Autodesk Inventor part; units mm, degrees
(part 2 of 2)
  line L319 (-28.6263, 18.3241) -> (-28.6263, 16.0044)
  line L320 (-28.6263, 16.0044) -> (-25.6449, 16.0044)
  line L321 (-25.6449, 18.3241) -> (-28.6263, 18.3241)
  line L322 (-29.7503, 19.4482) -> (-24.5209, 19.4482)
  line L323 (-29.5884, 13.8513) -> (-27.9357, 13.8513)
  line L324 (-29.5884, 12.8808) -> (-29.5884, 13.8513)
  line L325 (-29.7503, 14.8804) -> (-29.7503, 19.4482)
  line L326 (-26.6942, 13.8513) -> (-19.7097, 13.8513)
  line L327 (-23.8, 11.9101) -> (-23.8, 12.8808)
  line L328 (-25.8364, 11.9101) -> (-23.8, 11.9101)
  line L329 (-24.7124, 10.786) -> (-24.7124, 8.4664)
  line L330 (-21.731, 8.4664) -> (-21.731, 10.786)
  line L331 (-24.7124, 8.4664) -> (-21.731, 8.4664)
  line L332 (-21.731, 10.786) -> (-24.7124, 10.786)
  line L333 (-26.6942, 14.8804) -> (-26.6942, 13.8513)
  line L334 (-24.5209, 14.8804) -> (-26.6942, 14.8804)
  line L335 (-20.607, 11.9101) -> (-20.607, 7.3423)
  line L336 (-20.607, 7.3423) -> (-25.8364, 7.3423)
  line L337 (-25.8364, 7.3423) -> (-25.8364, 11.9101)
  line L338 (-27.9357, 14.8804) -> (-29.7503, 14.8804)
  line L339 (-37.8438, 41.8417) -> (-37.8438, 39.522)
  line L340 (-41.854, 38.3672) -> (-47.0835, 38.3672)
  line L341 (-45.9594, 39.4913) -> (-42.9781, 39.4913)
  line L342 (-42.9781, 39.4913) -> (-42.9781, 41.8109)
  line L343 (-39.6887, 44.9654) -> (-33.9003, 44.9654)
  line L344 (-43.779, 42.935) -> (-41.854, 42.935)
  line L345 (-42.9781, 41.8109) -> (-45.9594, 41.8109)
  line L346 (-47.8027, 44.9654) -> (-40.8666, 44.9654)
  line L347 (-43.779, 43.9948) -> (-43.779, 42.935)
  line L348 (-44.8621, 42.935) -> (-44.8621, 43.9948)
  line L349 (-47.0835, 42.935) -> (-44.8621, 42.935)
  line L350 (-44.8621, 43.9948) -> (-47.8027, 43.9948)
  line L351 (-45.9594, 41.8109) -> (-45.9594, 39.4913)
  line L352 (-47.0835, 38.3672) -> (-47.0835, 42.935)
  line L353 (-35.553, 43.9948) -> (-35.553, 42.9657)
  line L354 (-40.8666, 44.9654) -> (-40.8666, 45.9361)
  line L355 (-41.854, 42.935) -> (-41.854, 38.3672)
  line L356 (-40.8666, 45.9361) -> (-42.8818, 45.9361)
  line L357 (-47.8027, 43.9948) -> (-47.8027, 44.9654)
  line L358 (-38.9678, 38.398) -> (-38.9678, 42.9657)
  line L359 (-34.8624, 39.522) -> (-34.8624, 41.8417)
  line L360 (-34.8624, 41.8417) -> (-37.8438, 41.8417)
  line L361 (-37.8438, 39.522) -> (-34.8624, 39.522)
  line L362 (-33.7384, 38.398) -> (-38.9678, 38.398)
  line L363 (-33.9003, 43.9948) -> (-35.553, 43.9948)
  line L364 (-33.9003, 44.9654) -> (-33.9003, 43.9948)
  line L365 (-33.7384, 42.9657) -> (-33.7384, 38.398)
  line L366 (-36.7945, 43.9948) -> (-43.779, 43.9948)
  line L367 (-39.6887, 45.9361) -> (-39.6887, 44.9654)
  line L368 (-37.6523, 45.9361) -> (-39.6887, 45.9361)
  line L369 (-38.7764, 47.0601) -> (-38.7764, 49.3798)
  line L370 (-41.7577, 49.3798) -> (-41.7577, 47.0601)
  line L371 (-38.7764, 49.3798) -> (-41.7577, 49.3798)
  line L372 (-41.7577, 47.0601) -> (-38.7764, 47.0601)
  line L373 (-36.7945, 42.9657) -> (-36.7945, 43.9948)
  line L374 (-38.9678, 42.9657) -> (-36.7945, 42.9657)
  line L375 (-42.8818, 45.9361) -> (-42.8818, 50.5038)
  line L376 (-42.8818, 50.5038) -> (-37.6523, 50.5038)
  line L377 (-37.6523, 50.5038) -> (-37.6523, 45.9361)
  line L378 (-35.553, 42.9657) -> (-33.7384, 42.9657)
  line L379 (-40.5846, 75.534) -> (-40.5846, 13.366) construction
  line L380 (-23.2199, 44.9654) -> (-23.2199, 45.9361)
  line L381 (-23.2199, 45.9361) -> (-25.235, 45.9361)
  line L382 (-19.1478, 43.9948) -> (-26.1323, 43.9948)
  line L383 (-24.111, 47.0601) -> (-21.1296, 47.0601)
  line L384 (-20.0056, 45.9361) -> (-22.042, 45.9361)
  line L385 (-24.111, 49.3798) -> (-24.111, 47.0601)
  line L386 (-25.235, 45.9361) -> (-25.235, 50.5038)
  line L387 (-21.1296, 47.0601) -> (-21.1296, 49.3798)
  line L388 (-21.1296, 49.3798) -> (-24.111, 49.3798)
  line L389 (-25.235, 50.5038) -> (-20.0056, 50.5038)
  line L390 (-20.0056, 50.5038) -> (-20.0056, 45.9361)
  line L391 (-22.042, 45.9361) -> (-22.042, 44.9654)
  line L392 (-24.2073, 38.3672) -> (-29.4368, 38.3672)
  line L393 (-28.3127, 39.4913) -> (-25.3314, 39.4913)
  line L394 (-25.3314, 39.4913) -> (-25.3314, 41.8109)
  line L395 (-26.1323, 42.935) -> (-24.2073, 42.935)
  line L396 (-25.3314, 41.8109) -> (-28.3127, 41.8109)
  line L397 (-30.156, 44.9654) -> (-23.2199, 44.9654)
  line L398 (-27.2154, 42.935) -> (-27.2154, 43.9948)
  line L399 (-30.156, 43.9948) -> (-30.156, 44.9654)
  line L400 (-27.2154, 43.9948) -> (-30.156, 43.9948)
  line L401 (-29.4368, 42.935) -> (-27.2154, 42.935)
  line L402 (-28.3127, 41.8109) -> (-28.3127, 39.4913)
  line L403 (-29.4368, 38.3672) -> (-29.4368, 42.935)
  line L404 (-26.1323, 43.9948) -> (-26.1323, 42.935)
  line L405 (-20.1971, 41.8417) -> (-20.1971, 39.522)
  line L406 (-22.042, 44.9654) -> (-16.2536, 44.9654)
  line L407 (-17.9063, 43.9948) -> (-17.9063, 42.9657)
  line L408 (-24.2073, 42.935) -> (-24.2073, 38.3672)
  line L409 (-21.3211, 38.398) -> (-21.3211, 42.9657)
  line L410 (-21.3211, 42.9657) -> (-19.1478, 42.9657)
  line L411 (-19.1478, 42.9657) -> (-19.1478, 43.9948)
  line L412 (-16.2536, 44.9654) -> (-16.2536, 43.9948)
  line L413 (-16.2536, 43.9948) -> (-17.9063, 43.9948)
  line L414 (-17.2157, 41.8417) -> (-20.1971, 41.8417)
  line L415 (-17.9063, 42.9657) -> (-16.0917, 42.9657)
  line L416 (-20.1971, 39.522) -> (-17.2157, 39.522)
  line L417 (-16.0917, 38.398) -> (-21.3211, 38.398)
  line L418 (-16.0917, 42.9657) -> (-16.0917, 38.398)
  line L419 (-17.2157, 39.522) -> (-17.2157, 41.8417)
  spline S0 degree 2 poles (-50.3948, 78.6019) (-50.3948, 77.8197) (-50.9135, 76.4941) (-51.3498, 76.0495) knots 0 0 0 1 2 2 2
  spline S1 degree 2 poles (-51.3498, 76.0495) (-51.8027, 75.5802) (-52.9389, 75.0945) (-53.6222, 75.0945) knots 0 0 0 1 2 2 2
  spline S2 degree 2 poles (-53.6222, 75.0945) (-54.3056, 75.0945) (-55.4336, 75.5555) (-55.8617, 76.0166) knots 0 0 0 1 2 2 2
  spline S3 degree 2 poles (-55.8617, 76.0166) (-56.3887, 76.5682) (-56.9815, 78.4207) (-56.9815, 79.771) knots 0 0 0 1 2 2 2
  spline S4 degree 2 poles (-56.9815, 79.771) (-56.9815, 81.0966) (-56.4381, 83.229) (-55.87, 84.0195) knots 0 0 0 1 2 2 2
  spline S5 degree 2 poles (-55.87, 84.0195) (-55.3183, 84.7934) (-53.5728, 85.6579) (-52.4284, 85.6579) knots 0 0 0 1 2 2 2
  spline S6 degree 2 poles (-52.4284, 85.6579) (-52.0908, 85.6579) (-51.498, 85.592) (-51.2757, 85.5179) knots 0 0 0 1 2 2 2
  line L420 (-51.2757, 85.5179) -> (-51.2757, 84.2088)
  line L421 (-51.2757, 84.2088) -> (-51.3334, 84.2088)
  spline S7 degree 2 poles (-51.3334, 84.2088) (-51.5227, 84.3076) (-52.2143, 84.4805) (-52.6095, 84.4805) knots 0 0 0 1 2 2 2
  spline S8 degree 2 poles (-52.6095, 84.4805) (-53.8775, 84.4805) (-55.4336, 82.768) (-55.5818, 81.0884) knots 0 0 0 1 2 2 2
  spline S9 degree 2 poles (-55.5818, 81.0884) (-55.096, 81.4259) (-54.0751, 81.7964) (-53.4658, 81.7964) knots 0 0 0 1 2 2 2
  spline S10 degree 2 poles (-53.4658, 81.7964) (-52.873, 81.7964) (-51.9838, 81.5577) (-51.498, 81.1954) knots 0 0 0 1 2 2 2
  spline S11 degree 2 poles (-51.498, 81.1954) (-50.9382, 80.7755) (-50.3948, 79.4746) (-50.3948, 78.6019) knots 0 0 0 1 2 2 2
  spline S12 degree 2 poles (-51.778, 78.5442) (-51.778, 79.17) (-52.1073, 80.018) (-52.4696, 80.3144) knots 0 0 0 1 2 2 2
  spline S13 degree 2 poles (-52.4696, 80.3144) (-52.7413, 80.5285) (-53.4164, 80.6685) (-53.7704, 80.6685) knots 0 0 0 1 2 2 2
  spline S14 degree 2 poles (-53.7704, 80.6685) (-54.248, 80.6685) (-55.1454, 80.3803) (-55.5818, 80.1086) knots 0 0 0 1 2 2 2
  spline S15 degree 2 poles (-55.5818, 80.1086) (-55.59, 79.9604) (-55.6065, 79.6805) (-55.6065, 79.4664) knots 0 0 0 1 2 2 2
  spline S16 degree 2 poles (-55.6065, 79.4664) (-55.6065, 78.4125) (-55.1948, 77.1199) (-54.882, 76.7823) knots 0 0 0 1 2 2 2
  spline S17 degree 2 poles (-54.882, 76.7823) (-54.5938, 76.4612) (-53.968, 76.206) (-53.614, 76.206) knots 0 0 0 1 2 2 2
  spline S18 degree 2 poles (-53.614, 76.206) (-52.7907, 76.206) (-51.778, 77.3751) (-51.778, 78.5442) knots 0 0 0 1 2 2 2
  spline S19 degree 2 poles (-13.1052, 10.4678) (-13.1052, 11.2499) (-12.5865, 12.5755) (-12.1502, 13.0201) knots 0 0 0 1 2 2 2
  spline S20 degree 2 poles (-12.1502, 13.0201) (-11.6973, 13.4894) (-10.5611, 13.9752) (-9.8778, 13.9752) knots 0 0 0 1 2 2 2
  spline S21 degree 2 poles (-9.8778, 13.9752) (-9.1944, 13.9752) (-8.0664, 13.5141) (-7.6383, 13.053) knots 0 0 0 1 2 2 2
  spline S22 degree 2 poles (-7.6383, 13.053) (-7.1113, 12.5014) (-6.5185, 10.6489) (-6.5185, 9.2986) knots 0 0 0 1 2 2 2
  spline S23 degree 2 poles (-6.5185, 9.2986) (-6.5185, 7.973) (-7.0619, 5.8406) (-7.63, 5.0502) knots 0 0 0 1 2 2 2
  spline S24 degree 2 poles (-7.63, 5.0502) (-8.1817, 4.2763) (-9.9272, 3.4117) (-11.0716, 3.4117) knots 0 0 0 1 2 2 2
  spline S25 degree 2 poles (-11.0716, 3.4117) (-11.4092, 3.4117) (-12.002, 3.4776) (-12.2243, 3.5517) knots 0 0 0 1 2 2 2
  line L422 (-12.2243, 3.5517) -> (-12.2243, 4.8608)
  line L423 (-12.2243, 4.8608) -> (-12.1666, 4.8608)
  spline S26 degree 2 poles (-12.1666, 4.8608) (-11.9773, 4.762) (-11.2857, 4.5891) (-10.8905, 4.5891) knots 0 0 0 1 2 2 2
  spline S27 degree 2 poles (-10.8905, 4.5891) (-9.6225, 4.5891) (-8.0664, 6.3017) (-7.9182, 7.9813) knots 0 0 0 1 2 2 2
  spline S28 degree 2 poles (-7.9182, 7.9813) (-8.404, 7.6437) (-9.4249, 7.2732) (-10.0342, 7.2732) knots 0 0 0 1 2 2 2
  spline S29 degree 2 poles (-10.0342, 7.2732) (-10.627, 7.2732) (-11.5162, 7.512) (-12.002, 7.8742) knots 0 0 0 1 2 2 2
  spline S30 degree 2 poles (-12.002, 7.8742) (-12.5618, 8.2941) (-13.1052, 9.595) (-13.1052, 10.4678) knots 0 0 0 1 2 2 2
  spline S31 degree 2 poles (-11.722, 10.5254) (-11.722, 9.8997) (-11.3927, 9.0516) (-11.0304, 8.7552) knots 0 0 0 1 2 2 2
  spline S32 degree 2 poles (-11.0304, 8.7552) (-10.7587, 8.5411) (-10.0836, 8.4012) (-9.7296, 8.4012) knots 0 0 0 1 2 2 2
  spline S33 degree 2 poles (-9.7296, 8.4012) (-9.252, 8.4012) (-8.3546, 8.6893) (-7.9182, 8.961) knots 0 0 0 1 2 2 2
  spline S34 degree 2 poles (-7.9182, 8.961) (-7.91, 9.1092) (-7.8935, 9.3892) (-7.8935, 9.6033) knots 0 0 0 1 2 2 2
  spline S35 degree 2 poles (-7.8935, 9.6033) (-7.8935, 10.6571) (-8.3052, 11.9498) (-8.618, 12.2873) knots 0 0 0 1 2 2 2
  spline S36 degree 2 poles (-8.618, 12.2873) (-8.9062, 12.6084) (-9.532, 12.8637) (-9.886, 12.8637) knots 0 0 0 1 2 2 2
  spline S37 degree 2 poles (-9.886, 12.8637) (-10.7093, 12.8637) (-11.722, 11.6945) (-11.722, 10.5254) knots 0 0 0 1 2 2 2
  spline S38 degree 2 poles (-13.1052, 10.4678) (-13.1052, 11.2499) (-12.5865, 12.5755) (-12.1502, 13.0201) knots 0 0 0 1 2 2 2
  spline S39 degree 2 poles (-12.1502, 13.0201) (-11.6973, 13.4894) (-10.5611, 13.9752) (-9.8778, 13.9752) knots 0 0 0 1 2 2 2
  spline S40 degree 2 poles (-9.8778, 13.9752) (-9.1944, 13.9752) (-8.0664, 13.5141) (-7.6383, 13.053) knots 0 0 0 1 2 2 2
  spline S41 degree 2 poles (-7.6383, 13.053) (-7.1113, 12.5014) (-6.5185, 10.6489) (-6.5185, 9.2986) knots 0 0 0 1 2 2 2
  spline S42 degree 2 poles (-6.5185, 9.2986) (-6.5185, 7.973) (-7.0619, 5.8406) (-7.63, 5.0502) knots 0 0 0 1 2 2 2
  spline S43 degree 2 poles (-7.63, 5.0502) (-8.1817, 4.2763) (-9.9272, 3.4117) (-11.0716, 3.4117) knots 0 0 0 1 2 2 2
  spline S44 degree 2 poles (-11.0716, 3.4117) (-11.4092, 3.4117) (-12.002, 3.4776) (-12.2243, 3.5517) knots 0 0 0 1 2 2 2
  line L424 (-12.2243, 3.5517) -> (-12.2243, 4.8608)
  line L425 (-12.2243, 4.8608) -> (-12.1666, 4.8608)
  spline S45 degree 2 poles (-12.1666, 4.8608) (-11.9773, 4.762) (-11.2857, 4.5891) (-10.8905, 4.5891) knots 0 0 0 1 2 2 2
  spline S46 degree 2 poles (-10.8905, 4.5891) (-9.6225, 4.5891) (-8.0664, 6.3017) (-7.9182, 7.9813) knots 0 0 0 1 2 2 2
  spline S47 degree 2 poles (-7.9182, 7.9813) (-8.404, 7.6437) (-9.4249, 7.2732) (-10.0342, 7.2732) knots 0 0 0 1 2 2 2
  spline S48 degree 2 poles (-10.0342, 7.2732) (-10.627, 7.2732) (-11.5162, 7.512) (-12.002, 7.8742) knots 0 0 0 1 2 2 2
  spline S49 degree 2 poles (-12.002, 7.8742) (-12.5618, 8.2941) (-13.1052, 9.595) (-13.1052, 10.4678) knots 0 0 0 1 2 2 2
  spline S50 degree 2 poles (-11.722, 10.5254) (-11.722, 9.8997) (-11.3927, 9.0516) (-11.0304, 8.7552) knots 0 0 0 1 2 2 2
  spline S51 degree 2 poles (-11.0304, 8.7552) (-10.7587, 8.5411) (-10.0836, 8.4012) (-9.7296, 8.4012) knots 0 0 0 1 2 2 2
  spline S52 degree 2 poles (-9.7296, 8.4012) (-9.252, 8.4012) (-8.3546, 8.6893) (-7.9182, 8.961) knots 0 0 0 1 2 2 2
  spline S53 degree 2 poles (-7.9182, 8.961) (-7.91, 9.1092) (-7.8935, 9.3892) (-7.8935, 9.6033) knots 0 0 0 1 2 2 2
  spline S54 degree 2 poles (-7.8935, 9.6033) (-7.8935, 10.6571) (-8.3052, 11.9498) (-8.618, 12.2873) knots 0 0 0 1 2 2 2
  spline S55 degree 2 poles (-8.618, 12.2873) (-8.9062, 12.6084) (-9.532, 12.8637) (-9.886, 12.8637) knots 0 0 0 1 2 2 2
  spline S56 degree 2 poles (-9.886, 12.8637) (-10.7093, 12.8637) (-11.722, 11.6945) (-11.722, 10.5254) knots 0 0 0 1 2 2 2
  spline S57 degree 2 poles (-50.3948, 78.6019) (-50.3948, 77.8197) (-50.9135, 76.4941) (-51.3498, 76.0495) knots 0 0 0 1 2 2 2
  spline S58 degree 2 poles (-51.3498, 76.0495) (-51.8027, 75.5802) (-52.9389, 75.0945) (-53.6222, 75.0945) knots 0 0 0 1 2 2 2
  spline S59 degree 2 poles (-53.6222, 75.0945) (-54.3056, 75.0945) (-55.4336, 75.5555) (-55.8617, 76.0166) knots 0 0 0 1 2 2 2
  spline S60 degree 2 poles (-55.8617, 76.0166) (-56.3887, 76.5682) (-56.9815, 78.4207) (-56.9815, 79.771) knots 0 0 0 1 2 2 2
  spline S61 degree 2 poles (-56.9815, 79.771) (-56.9815, 81.0966) (-56.4381, 83.229) (-55.87, 84.0195) knots 0 0 0 1 2 2 2
  spline S62 degree 2 poles (-55.87, 84.0195) (-55.3183, 84.7934) (-53.5728, 85.6579) (-52.4284, 85.6579) knots 0 0 0 1 2 2 2
  spline S63 degree 2 poles (-52.4284, 85.6579) (-52.0908, 85.6579) (-51.498, 85.592) (-51.2757, 85.5179) knots 0 0 0 1 2 2 2
  line L426 (-51.2757, 85.5179) -> (-51.2757, 84.2088)
  line L427 (-51.2757, 84.2088) -> (-51.3334, 84.2088)
  spline S64 degree 2 poles (-51.3334, 84.2088) (-51.5227, 84.3076) (-52.2143, 84.4805) (-52.6095, 84.4805) knots 0 0 0 1 2 2 2
  spline S65 degree 2 poles (-52.6095, 84.4805) (-53.8775, 84.4805) (-55.4336, 82.768) (-55.5818, 81.0884) knots 0 0 0 1 2 2 2
  spline S66 degree 2 poles (-55.5818, 81.0884) (-55.096, 81.4259) (-54.0751, 81.7964) (-53.4658, 81.7964) knots 0 0 0 1 2 2 2
  spline S67 degree 2 poles (-53.4658, 81.7964) (-52.873, 81.7964) (-51.9838, 81.5577) (-51.498, 81.1954) knots 0 0 0 1 2 2 2
  spline S68 degree 2 poles (-51.498, 81.1954) (-50.9382, 80.7755) (-50.3948, 79.4746) (-50.3948, 78.6019) knots 0 0 0 1 2 2 2
  spline S69 degree 2 poles (-51.778, 78.5442) (-51.778, 79.17) (-52.1073, 80.018) (-52.4696, 80.3144) knots 0 0 0 1 2 2 2
  spline S70 degree 2 poles (-52.4696, 80.3144) (-52.7413, 80.5285) (-53.4164, 80.6685) (-53.7704, 80.6685) knots 0 0 0 1 2 2 2
  spline S71 degree 2 poles (-53.7704, 80.6685) (-54.248, 80.6685) (-55.1454, 80.3803) (-55.5818, 80.1086) knots 0 0 0 1 2 2 2
  spline S72 degree 2 poles (-55.5818, 80.1086) (-55.59, 79.9604) (-55.6065, 79.6805) (-55.6065, 79.4664) knots 0 0 0 1 2 2 2
  spline S73 degree 2 poles (-55.6065, 79.4664) (-55.6065, 78.4125) (-55.1948, 77.1199) (-54.882, 76.7823) knots 0 0 0 1 2 2 2
  spline S74 degree 2 poles (-54.882, 76.7823) (-54.5938, 76.4612) (-53.968, 76.206) (-53.614, 76.206) knots 0 0 0 1 2 2 2
  spline S75 degree 2 poles (-53.614, 76.206) (-52.7907, 76.206) (-51.778, 77.3751) (-51.778, 78.5442) knots 0 0 0 1 2 2 2
  point P0 (-53.7479, 68.8958)
  point P1 (-9.7521, 20.0042)
  point P2 (-41.8348, 101.4209)
  point P3 (-53.7479, 68.8958)
  point P4 (-9.7521, 20.0042)
  point P5 (-1, 6.9835)
  point P6 (-22.9154, 75.534)
  point P7 (-94.7005, 61.8998)
  point P8 (-94.7005, 61.8998)
  point P9 (-22.9154, 75.534)
  point P10 (-22.9154, 75.534)
  point P11 (-22.9154, 13.366)
  point P12 (-22.9154, 13.366)
  point P13 (-22.9154, 13.366)
  point P14 (-40.5734, 44.4801)
  point P15 (-40.5734, 44.4801)
  point P16 (-22.9266, 44.4801)
  point P17 (-22.9266, 44.4801)
  point P18 (-22.9266, 44.4801)
  dimension "d155" = 8.4153
  dimension "d157" = 0.508
  dimension "d158" = 4.5466
  dimension "d159" = 0.508
  dimension "d160" = 4.5466
  constraints: 814 end point, 50 parallel, 20 perpendicular, 14 horizontal, 5 midpoint, 2 symmetric about line, 1 vertical, 14 other
  measures "d155" distance of L174.end L172.start
  measures "d157" distance between parallel lines of L7 L173
  measures "d158" distance from line of point (-1, 6.983) L172
  measures "d159" distance between parallel lines of L6 L168
  measures "d160" distance between parallel lines of L4 L171
extrude "Extrusion20" add sketch "Sketch17" along normal blind 0.4 contours L48 L49 L73 L71 L76 L69 L86 L79 L85 L67 L62 L68 L84 L80 L87 L77 L82 L60 L55 L61 L81 L78 L83 L70 L75 L72 L74 L50 | L88 L89 L113 L111 L116 L109 L126 L119 L125 L107 L102 L108 L124 L120 L127 L117 L122 L100 L95 L101 L121 L118 L123 L110 L115 L112 L114 L90 | L128 L129 L153 L151 L156 L149 L166 L159 L165 L147 L142 L148 L164 L160 L167 L157 L162 L140 L135 L141 L161 L158 L163 L150 L155 L152 L154 L130 | L219 L225 L226 L229 L230 L231 L234 L232 L233 L249 L247 L248 L257 L256 L237 L238 L239 L235 L246 L245 L244 L241 L255 L254 L258 L228 L223 L224 | L260 L272 L269 L268 L270 L277 L266 L274 L276 L295 L296 L297 L288 L287 L263 L284 L283 L273 L298 L285 L282 L278 L294 L293 L286 L267 L264 L275 | L300 L312 L309 L308 L310 L317 L306 L314 L316 L335 L336 L337 L328 L327 L303 L324 L323 L313 L338 L325 L322 L318 L334 L333 L326 L307 L304 L315 | L340 L352 L349 L348 L350 L357 L346 L354 L356 L375 L376 L377 L368 L367 L343 L364 L363 L353 L378 L365 L362 L358 L374 L373 L366 L347 L344 L355 | L380 L381 L386 L389 L390 L384 L391 L406 L412 L413 L407 L415 L418 L417 L409 L410 L411 L382 L404 L395 L408 L392 L403 L401 L398 L400 L399 L397 | S0 S1 S2 S3 S4 S5 S6 L420 L421 S7 S8 S9 S10 S11 | S19 S20 S21 S22 S23 S24 S25 L422 L423 S26 S27 S28 S29 S30 bodies 2
sketch "Sketch18" plane through (0, 0, -0.2) normal (0, 0, -1) x (-1, 0, 0)
  line L0 (0, 0) -> (-63.5, 0)
  line L1 (-63.5, 0) -> (-63.5, 88.9)
  line L2 (-63.5, 88.9) -> (0, 88.9)
  line L3 (0, 88.9) -> (0, 0)
  constraints: 8 end point, 2 parallel, 1 horizontal, 1 perpendicular
extrude "Extrusion21" add sketch "Sketch18" along normal blind 0.4 bodies 3
fillet "Fillet2" radius 3.175 8 edges at (63.5, 0, 0.2) (63.5, 88.9, 0.2) (0, 0, 0.2) (0, 88.9, 0.2) (63.5, 0, -0.3) (63.5, 88.9, -0.3) (0, 0, -0.3) (0, 88.9, -0.3)
extrude "Extrusion22" cut sketch "Sketch17" along normal blind 0.4 contours L48 L49 L73 L71 L76 L69 L86 L79 L85 L67 L62 L68 L84 L80 L87 L77 L82 L60 L55 L61 L81 L78 L83 L70 L75 L72 L74 L50 | L88 L89 L113 L111 L116 L109 L126 L119 L125 L107 L102 L108 L124 L120 L127 L117 L122 L100 L95 L101 L121 L118 L123 L110 L115 L112 L114 L90 | L128 L129 L153 L151 L156 L149 L166 L159 L165 L147 L142 L148 L164 L160 L167 L157 L162 L140 L135 L141 L161 L158 L163 L150 L155 L152 L154 L130 | L219 L225 L226 L229 L230 L231 L234 L232 L233 L249 L247 L248 L257 L256 L237 L238 L239 L235 L246 L245 L244 L241 L255 L254 L258 L228 L223 L224 | L260 L272 L269 L268 L270 L277 L266 L274 L276 L295 L296 L297 L288 L287 L263 L284 L283 L273 L298 L285 L282 L278 L294 L293 L286 L267 L264 L275 | L300 L312 L309 L308 L310 L317 L306 L314 L316 L335 L336 L337 L328 L327 L303 L324 L323 L313 L338 L325 L322 L318 L334 L333 L326 L307 L304 L315 | L340 L352 L349 L348 L350 L357 L346 L354 L356 L375 L376 L377 L368 L367 L343 L364 L363 L353 L378 L365 L362 L358 L374 L373 L366 L347 L344 L355 | L380 L381 L386 L389 L390 L384 L391 L406 L412 L413 L407 L415 L418 L417 L409 L410 L411 L382 L404 L395 L408 L392 L403 L401 L398 L400 L399 L397 | S0 S1 S2 S3 S4 S5 S6 L420 L421 S7 S8 S9 S10 S11 | S19 S20 S21 S22 S23 S24 S25 L422 L423 S26 S27 S28 S29 S30 bodies 3
